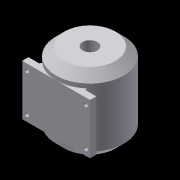
# Autodesk Inventor part: Motor
Saved by Autodesk Inventor 2020 (Build 240168000, 168)
## iProperties
Created: 2019-08-12
Part Number: Motor
Document SubType Name: Modeling
Designer: Administrator
Density: 1 g/cm^3
Mass: 3.61536 g
Surface Area: 14.4035 cm^2
Volume: 3.61536 cm^3
Material: 一般
Appearance: 冷白色
Author: Administrator
Autodesk Inventor part; units mm, degrees
ref_plane "YZ Plane" through (0, 0, 0) normal (1, 0, 0) x (0, 1, 0)
ref_plane "XZ Plane" through (0, 0, 0) normal (0, 1, 0) x (-1, 0, 0)
ref_plane "XY Plane" through (0, 0, 0) normal (0, 0, 1) x (1, 0, 0)
sketch "Sketch1" plane through (0, 0, 0) normal (0, 0, 1) x (1, 0, 0)
  arc A0 (5.2535, -6.0994) -> (-5.2535, -6.0994) centre (0, 0) ccw
  line L0 (0, 0) -> (0, -8.05) construction
  line L1 (0, -8.05) -> (8.05, -8.05)
  line L2 (8.05, -8.05) -> (8.05, -6.55)
  line L3 (8.05, -6.55) -> (5.5137, -6.55)
  line L4 (0, 0) -> (4.025, -6.9715) construction
  line L5 (5.5137, -6.55) -> (5.2535, -6.0994)
  line L6 (0, 0) -> (8.05, 0) construction
  line L7 (0, -8.05) -> (-8.05, -8.05)
  line L8 (-8.05, -8.05) -> (-8.05, -6.55)
  line L9 (-8.05, -6.55) -> (-5.5137, -6.55)
  line L10 (-5.5137, -6.55) -> (-5.2535, -6.0994)
  dimension "d0" = 16.1
  dimension "d1" = 30
  dimension "d2" = 1.5
  dimension "d3" = 1.5
  constraints: 22 end point, 4 parallel, 4 symmetric about line, 3 point on circle, 2 perpendicular, 1 centre point, 1 tangent, 1 vertical, 1 other
  measures "d0" diameter of A0
  measures "d1" angle of L4 L0
  measures "d2" distance between parallel lines of L5 L4
  measures "d3" distance of L1.end L2.end
extrude "Extrusion1" add sketch "Sketch1" along normal mid plane 12
sketch "Sketch2" plane through (0, 0, 0) normal (0, 0, 1) x (1, 0, 0)
  arc A0 (5.2535, -6.0994) -> (-5.2535, -6.0994) centre (0, 0) ccw projected
  circle A1 centre (0, 0) radius 8.05
  point P0 (4.8598, -6.4175)
  constraints: 1 centre point, 1 coincident, 1 concentric
extrude "Extrusion2" add sketch "Sketch2" along normal mid plane 18
chamfer "Chamfer1" distance 2 angle 45 2 edges at (-8.05, 0, 9) (-8.05, 0, -9)
sketch "Sketch3" plane through (0, 0, 9) normal (0, 0, 1) x (1, 0, 0)
  circle A0 centre (0, 0) radius 6.05 projected
  circle A1 centre (0, 0) radius 1.75
  dimension "d11" = 3.5
  constraints: 1 centre point, 1 coincident
  measures "d11" diameter of A1
extrude "Extrusion3" cut sketch "Sketch3" against normal blind 4 contours A1
sketch "Sketch4" plane through (-8.05, -8.05, 6) normal (0, -1, 0) x (1, 0, 0)
  line L0 (0, -12) -> (0, 0) projected
  line L1 (16.1, -12) -> (16.1, 0) projected
  line L2 (16.1, 0) -> (8.05, 0) projected
  line L3 (8.05, 0) -> (8.05, -12) construction
  line L4 (0, -6) -> (16.1, -6) construction
  line L5 (1.05, -1.5) -> (15.05, -1.5) construction
  line L6 (15.05, -1.5) -> (15.05, -10.5) construction
  line L7 (15.05, -10.5) -> (1.05, -10.5) construction
  line L8 (1.05, -10.5) -> (1.05, -1.5) construction
  circle A0 centre (1.05, -1.5) radius 0.5
  circle A1 centre (15.05, -1.5) radius 0.5
  circle A2 centre (1.05, -10.5) radius 0.5
  circle A3 centre (15.05, -10.5) radius 0.5
  dimension "d14" = 9
  dimension "d15" = 4.5
  dimension "d16" = 14
  dimension "d17" = 7
  dimension "d18" = 1
  constraints: 12 end point, 4 centre point, 4 coincident, 3 equal radius, 2 midpoint, 2 parallel, 2 perpendicular, 1 horizontal
  measures "d14" distance of L7.end L5.start
  measures "d15" distance between parallel lines of L5 L4
  measures "d16" distance between parallel lines of L6 L8
  measures "d17" distance between parallel lines of L8 L3
  measures "d18" diameter of A0
extrude "Extrusion4" cut sketch "Sketch4" against normal up to surface (1.5 mm away)
